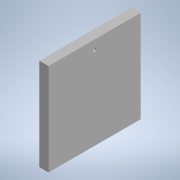
# Autodesk Inventor part: TMP_fix_plate
Saved by Autodesk Inventor 2022 (Build 260153000, 153)
## iProperties
Created: 2022-06-22
Part Number: TMP_fix_plate
Material: Generic
Document SubType Name: Modeling
Designer: dovalle
Density: 1 g/cm^3
Appearance: Default
Author: dovalle
Autodesk Inventor part; units mm, degrees
ref_plane "YZ Plane" through (0, 0, 0) normal (1, 0, 0) x (0, 1, 0)
ref_plane "XZ Plane" through (0, 0, 0) normal (0, 1, 0) x (-1, 0, 0)
ref_plane "XY Plane" through (0, 0, 0) normal (0, 0, 1) x (1, 0, 0)
sketch "Sketch1" plane through (0, 0, 0) normal (1, 0, 0) x (0, 1, 0)
  line L0 (0, 100) -> (-100, 100)
  line L1 (-100, 100) -> (-100, -100)
  line L2 (-100, -100) -> (100, -100)
  line L3 (100, -100) -> (100, 100)
  line L4 (100, 100) -> (0, 100)
  point P0 (0, 0)
  dimension "d1" = 100
  dimension "d2" = 200
  dimension "d3" = 200
  dimension "d4" = 200
  constraints: 10 end point, 2 perpendicular, 1 point on line
  measures "d1" distance of L0.start L0.end
  measures "d2" distance of L0.end L1.end
  measures "d3" distance of L1.end L2.end
  measures "d4" distance of L2.end L3.end
extrude "Extrusion1" add sketch "Sketch1" along normal blind 20
sketch "Sketch2" plane through (0, 0, 0) normal (-1, 0, 0) x (0, 0, 1)
  circle A0 centre (-56.5685, 56.5685) radius 4
  point P0 (0, 0)
  dimension "d11" = 8
  constraints: 1 centre point
  measures "d11" diameter of A0
extrude "Extrusion2" cut sketch "Sketch2" against normal blind 20
pattern_circular "Circular Pattern1" count 4 over 360 about axis through (-10, 0, 0) along (1, 0, 0) of "Extrusion2"
sketch "Sketch3" plane through (0, 0, 0) normal (-1, 0, 0) x (0, 0, 1)
  circle A0 centre (-56.5685, -56.5685) radius 4 projected
  circle A1 centre (56.5685, -56.5685) radius 4 projected
  circle A2 centre (0, -56.5685) radius 4
  point P0 (0, 0)
  dimension "d17" = 8
  constraints: 1 centre point
  measures "d17" diameter of A2
extrude "Extrusion3" cut sketch "Sketch3" against normal blind 20 contours A2
body "Solid1"
